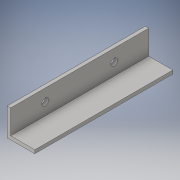
# Autodesk Inventor part: Ls in motor tensioner
Saved by Autodesk Inventor 2016 SP2 (Build 200236200, 236)
## iProperties
Created: 2018-02-02
Part Number: Ls in motor tensioner
Material: Generic
Document SubType Name: Modeling
Designer: CAD
Density: 1 g/cm^3
Appearance: Default
Author: CAD
Autodesk Inventor part; units mm, degrees
ref_plane "YZ Plane" through (0, 0, 0) normal (1, 0, 0) x (0, 1, 0)
ref_plane "XZ Plane" through (0, 0, 0) normal (0, 1, 0) x (-1, 0, 0)
ref_plane "XY Plane" through (0, 0, 0) normal (0, 0, 1) x (1, 0, 0)
sketch "Sketch1" plane through (0, 0, 0) normal (0, 0, 1) x (1, 0, 0)
  line L0 (0, 0) -> (-25.4, 0)
  line L1 (-25.4, 0) -> (-25.4, 25.4)
  line L2 (0, 3.175) -> (-22.225, 3.175)
  line L3 (-22.225, 3.175) -> (-22.225, 25.4)
  line L4 (0, 3.175) -> (0, 0)
  line L5 (-25.4, 25.4) -> (-22.225, 25.4)
  dimension "d0" = 25.4
  dimension "d2" = 25.4
  dimension "d3" = 3.175
  constraints: 12 end point, 2 vertical, 1 horizontal, 1 perpendicular, 1 other
  measures "d0" distance of L0.start L0.end
  measures "d2" distance of L0.end L1.end
  measures "d3" distance between parallel lines of L0 L2
extrude "Extrusion1" add sketch "Sketch1" along normal blind 127
sketch "Sketch2" plane through (-22.225, 3.175, 0) normal (1, 0, 0) x (0, 0, -1)
  line L0 (0, 22.225) -> (-127, 22.225) projected
  line L1 (-127, 0) -> (-127, 22.225) projected
  point P0 (0, -3.175)
  point P1 (-95.25, 11.1125)
  point P2 (-31.75, 11.1125)
  dimension "d6" = 11.1125
  dimension "d7" = 11.1125
  dimension "d8" = 63.5
  dimension "d9" = 31.75
  measures "d6" distance from line of L0 point (-95.25, 11.112)
  measures "d7" distance from line of L0 point (-31.75, 11.112)
  measures "d8" distance of point (-31.75, 11.112) point (-95.25, 11.112)
  measures "d9" distance from line of L1 point (-95.25, 11.112)
hole "Hole1" at (-22.225, 14.2875, 95.25) at (-22.225, 14.2875, 31.75) direction (-1, 0, 0) diameter 6.35 depth 25.4 tip angle 118
body "Solid1"
